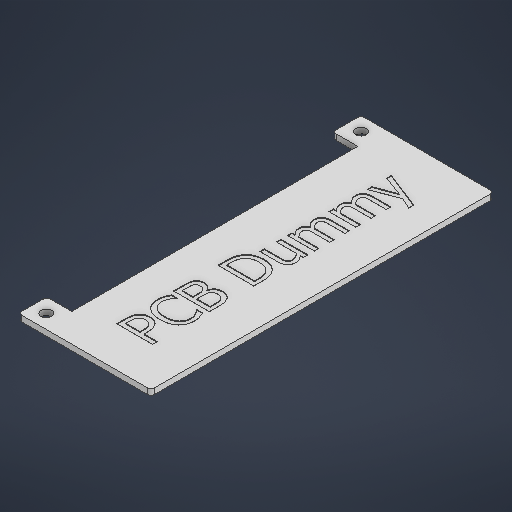
# Autodesk Inventor part: PCBDummy
Saved by Autodesk Inventor 2027 (Build 310192000, 192)
## iProperties
Created: 2026-09-26
Part Number: PCBDummy
Material: Všeobecné
Document SubType Name: Modeling
Designer: Vadim
Density: 1 g/cm^3
Appearance: Výchozí
Author: Vadim
Autodesk Inventor part; units mm, degrees
ref_plane "YZ Plane" through (0, 0, 0) normal (1, 0, 0) x (0, 1, 0)
ref_plane "XZ Plane" through (0, 0, 0) normal (0, 1, 0) x (-1, 0, 0)
ref_plane "XY Plane" through (0, 0, 0) normal (0, 0, 1) x (1, 0, 0)
sketch "Náčrt1" plane through (0, 0, 0) normal (0, 1, 0) x (-1, 0, 0)
  circle A0 centre (3.1, 43.9) radius 1.5
  circle A1 centre (3.1, -43.9) radius 1.5
  line L0 (7, 46.8) -> (7, 40.9)
  line L1 (6, 39.9) -> (0, 39.9)
  line L2 (0, 39.9) -> (0, -39.9)
  line L3 (0, -39.9) -> (6, -39.9)
  line L4 (7, -40.9) -> (7, -46.8)
  line L5 (6, -47.8) -> (-29, -47.8)
  line L6 (-30, -46.8) -> (-30, 46.8)
  line L7 (-29, 47.8) -> (6, 47.8)
  arc A2 (7, 46.8) -> (6, 47.8) centre (6, 46.8) ccw
  arc A3 (6, -47.8) -> (7, -46.8) centre (6, -46.8) ccw
  arc A4 (7, -40.9) -> (6, -39.9) centre (6, -40.9) ccw
  arc A5 (6, 39.9) -> (7, 40.9) centre (6, 40.9) ccw
  line L8 (0, 0) -> (-30, 0)
  arc A6 (-29, 47.8) -> (-30, 46.8) centre (-29, 46.8) ccw
  arc A7 (-30, -46.8) -> (-29, -47.8) centre (-29, -46.8) ccw
  dimension "d1" = 3
  dimension "d2" = 3
  dimension "d3" = 3.9
  dimension "d4" = 3.9
  dimension "d5" = 4
  dimension "d6" = 3.9
  dimension "d7" = 3.9
  dimension "d8" = 4
  dimension "d9" = 1
  dimension "d10" = 87.8
  dimension "d11" = 37
  dimension "d12" = 1
  dimension "d19" = 30
  constraints: 18 end point, 12 point on circle, 12 tangent, 8 centre point, 6 perpendicular, 4 equal radius, 2 midpoint, 1 coincident, 1 collinear
  measures "d1" diameter of A0
  measures "d2" diameter of A1
  measures "d3" distance from line of L0 A0.centre
  measures "d4" distance from line of L7 A0.centre
  measures "d5" distance from line of L1 A0.centre
  measures "d6" distance from line of L4 A1.centre
  measures "d7" distance from line of L5 A1.centre
  measures "d8" distance from line of A1.centre L3
  measures "d9" radius of A2
  measures "d10" distance of A1.centre A0.centre
  measures "d11" distance between parallel lines of L6 L4
  measures "d12" radius of A6
  measures "d19" distance between parallel lines of L6 L2
extrude "Vysunutí1" add sketch "Náčrt1" along normal blind 1.6
sketch "Náčrt2" plane through (0, 1.6, 0) normal (0, 1, 0) x (1, 0, 0)
  arc A0 (-6, -39.9) -> (-7, -40.9) centre (-6, -40.9) ccw projected
  line L0 (-7, -40.9) -> (-7, -46.8) projected
  arc A1 (-7, -46.8) -> (-6, -47.8) centre (-6, -46.8) ccw projected
  line L1 (-6, -47.8) -> (29, -47.8) projected
  arc A2 (29, -47.8) -> (30, -46.8) centre (29, -46.8) ccw projected
  line L2 (30, -46.8) -> (30, 46.8) projected
  arc A3 (30, 46.8) -> (29, 47.8) centre (29, 46.8) ccw projected
  line L3 (29, 47.8) -> (-6, 47.8) projected
  arc A4 (-6, 47.8) -> (-7, 46.8) centre (-6, 46.8) ccw projected
  line L4 (-7, 46.8) -> (-7, 40.9) projected
  arc A5 (-7, 40.9) -> (-6, 39.9) centre (-6, 40.9) ccw projected
  line L5 (-6, 39.9) -> (0, 39.9) projected
  line L6 (0, 39.9) -> (0, -39.9) projected
  line L7 (0, -39.9) -> (-6, -39.9) projected
  circle A6 centre (-3.1, 43.9) radius 1.5 projected
  circle A7 centre (-3.1, -43.9) radius 1.5 projected
  line L8 (1, -37.8) -> (1, 37.8) construction
  line L9 (1, 37.8) -> (22, 37.8) construction
  line L10 (22, 37.8) -> (22, -37.8) construction
  line L11 (22, -37.8) -> (1, -37.8) construction
  line L12 (0, 0) -> (30, 0) construction
  line L13 (11.5, -47.8) -> (11.5, 47.8) construction
  spline S0 degree 2 poles (12.2512, -30.2553) (12.8995, -30.2553) (14.0665, -30.7172) (14.4716, -31.1305) knots 0 0 0 1 2 2 2
  spline S1 degree 2 poles (14.4716, -31.1305) (14.9822, -31.6491) (15.5089, -33.0511) (15.5089, -34.1207) knots 0 0 0 1 2 2 2
  line L14 (15.5089, -34.1207) -> (15.5089, -35.2472)
  line L15 (15.5089, -35.2472) -> (19.2366, -35.2472)
  line L16 (19.2366, -35.2472) -> (19.2366, -36.5762)
  line L17 (19.2366, -36.5762) -> (9.2366, -36.5762)
  line L18 (9.2366, -36.5762) -> (9.2366, -34.064)
  spline S2 degree 2 poles (9.2366, -34.064) (9.2366, -33.1726) (9.5284, -31.9246) (9.8606, -31.4465) knots 0 0 0 1 2 2 2
  spline S3 degree 2 poles (9.8606, -31.4465) (10.2415, -30.8874) (11.4165, -30.2553) (12.2512, -30.2553) knots 0 0 0 1 2 2 2
  spline S4 degree 2 poles (12.2917, -31.641) (11.7731, -31.641) (11.0113, -31.9976) (10.7682, -32.3622) knots 0 0 0 1 2 2 2
  spline S5 degree 2 poles (10.7682, -32.3622) (10.5575, -32.6783) (10.3874, -33.5211) (10.3874, -34.1451) knots 0 0 0 1 2 2 2
  line L19 (10.3874, -34.1451) -> (10.3874, -35.2472)
  line L20 (10.3874, -35.2472) -> (14.3744, -35.2472)
  line L21 (14.3744, -35.2472) -> (14.3744, -34.3395)
  spline S6 degree 2 poles (14.3744, -34.3395) (14.3744, -33.5292) (14.1151, -32.5324) (13.7747, -32.2083) knots 0 0 0 1 2 2 2
  spline S7 degree 2 poles (13.7747, -32.2083) (13.4749, -31.9084) (12.7699, -31.641) (12.2917, -31.641) knots 0 0 0 1 2 2 2
  spline S8 degree 2 poles (19.4149, -25.0851) (19.4149, -26.0575) (18.7585, -27.7026) (18.1021, -28.3023) knots 0 0 0 1 2 2 2
  spline S9 degree 2 poles (18.1021, -28.3023) (17.4538, -28.9019) (15.5089, -29.5583) (14.2447, -29.5583) knots 0 0 0 1 2 2 2
  spline S10 degree 2 poles (14.2447, -29.5583) (12.9887, -29.5583) (11.1248, -28.9182) (10.436, -28.3104) knots 0 0 0 1 2 2 2
  spline S11 degree 2 poles (10.436, -28.3104) (9.7634, -27.7107) (9.0583, -26.0737) (9.0583, -25.0608) knots 0 0 0 1 2 2 2
  spline S12 degree 2 poles (9.0583, -25.0608) (9.0583, -24.5583) (9.2042, -23.675) (9.3177, -23.3023) knots 0 0 0 1 2 2 2
  spline S13 degree 2 poles (9.3177, -23.3023) (9.423, -22.9781) (9.7229, -22.3055) (9.9011, -21.9733) knots 0 0 0 1 2 2 2
  line L22 (9.9011, -21.9733) -> (11.5057, -21.9733)
  line L23 (11.5057, -21.9733) -> (11.5057, -22.0786)
  spline S14 degree 2 poles (11.5057, -22.0786) (11.3436, -22.2569) (10.8898, -22.8079) (10.671, -23.205) knots 0 0 0 1 2 2 2
  spline S15 degree 2 poles (10.671, -23.205) (10.4603, -23.5859) (10.1929, -24.4854) (10.1929, -25.0689) knots 0 0 0 1 2 2 2
  spline S16 degree 2 poles (10.1929, -25.0689) (10.1929, -25.7091) (10.7196, -26.8517) (11.222, -27.2812) knots 0 0 0 1 2 2 2
  spline S17 degree 2 poles (11.222, -27.2812) (11.7326, -27.7026) (13.2804, -28.1726) (14.2447, -28.1726) knots 0 0 0 1 2 2 2
  spline S18 degree 2 poles (14.2447, -28.1726) (15.2739, -28.1726) (16.7569, -27.6783) (17.2674, -27.2488) knots 0 0 0 1 2 2 2
  spline S19 degree 2 poles (17.2674, -27.2488) (17.7618, -26.8274) (18.2642, -25.701) (18.2642, -25.0689) knots 0 0 0 1 2 2 2
  spline S20 degree 2 poles (18.2642, -25.0689) (18.2642, -24.4935) (17.9806, -23.513) (17.7699, -23.1321) knots 0 0 0 1 2 2 2
  spline S21 degree 2 poles (17.7699, -23.1321) (17.5592, -22.7674) (17.1216, -22.2245) (16.9676, -22.0705) knots 0 0 0 1 2 2 2
  line L24 (16.9676, -22.0705) -> (16.9676, -21.9733)
  line L25 (16.9676, -21.9733) -> (18.5559, -21.9733)
  spline S22 degree 2 poles (18.5559, -21.9733) (18.7099, -22.3055) (18.9935, -22.889) (19.1232, -23.3023) knots 0 0 0 1 2 2 2
  spline S23 degree 2 poles (19.1232, -23.3023) (19.269, -23.7399) (19.4149, -24.4854) (19.4149, -25.0851) knots 0 0 0 1 2 2 2
  spline S24 degree 2 poles (16.1653, -13.9506) (16.9109, -13.9506) (18.0535, -14.5178) (18.4263, -14.9878) knots 0 0 0 1 2 2 2
  spline S25 degree 2 poles (18.4263, -14.9878) (18.8639, -15.5551) (19.2366, -16.8436) (19.2366, -17.8647) knots 0 0 0 1 2 2 2
  line L26 (19.2366, -17.8647) -> (19.2366, -20.7334)
  line L27 (19.2366, -20.7334) -> (9.2366, -20.7334)
  line L28 (9.2366, -20.7334) -> (9.2366, -18.0835)
  spline S26 degree 2 poles (9.2366, -18.0835) (9.2366, -17.0138) (9.3744, -15.9441) (9.6418, -15.4579) knots 0 0 0 1 2 2 2
  spline S27 degree 2 poles (9.6418, -15.4579) (9.9254, -14.9149) (10.8574, -14.4206) (11.4895, -14.4206) knots 0 0 0 1 2 2 2
  spline S28 degree 2 poles (11.4895, -14.4206) (12.1945, -14.4206) (13.3128, -15.1661) (13.6288, -15.8225) knots 0 0 0 1 2 2 2
  line L29 (13.6288, -15.8225) -> (13.6775, -15.8225)
  spline S29 degree 2 poles (13.6775, -15.8225) (13.9206, -14.9311) (15.2091, -13.9506) (16.1653, -13.9506) knots 0 0 0 1 2 2 2
  spline S30 degree 2 poles (16.222, -15.3363) (15.6548, -15.3363) (14.9254, -15.6605) (14.6661, -16.1467) knots 0 0 0 1 2 2 2
  spline S31 degree 2 poles (14.6661, -16.1467) (14.5041, -16.4627) (14.4068, -17.2083) (14.4068, -17.8971) knots 0 0 0 1 2 2 2
  line L30 (14.4068, -17.8971) -> (14.4068, -19.4044)
  line L31 (14.4068, -19.4044) -> (18.1021, -19.4044)
  line L32 (18.1021, -19.4044) -> (18.1021, -18.3266)
  spline S32 degree 2 poles (18.1021, -18.3266) (18.1021, -17.4514) (17.94, -16.4465) (17.6807, -16.0575) knots 0 0 0 1 2 2 2
  spline S33 degree 2 poles (17.6807, -16.0575) (17.4133, -15.6848) (16.7488, -15.3363) (16.222, -15.3363) knots 0 0 0 1 2 2 2
  spline S34 degree 2 poles (11.6759, -15.8063) (11.3193, -15.8063) (10.7844, -16.0494) (10.6305, -16.3169) knots 0 0 0 1 2 2 2
  spline S35 degree 2 poles (10.6305, -16.3169) (10.4522, -16.641) (10.3712, -17.4271) (10.3712, -18.1321) knots 0 0 0 1 2 2 2
  line L33 (10.3712, -18.1321) -> (10.3712, -19.4044)
  line L34 (10.3712, -19.4044) -> (13.2966, -19.4044)
  line L35 (13.2966, -19.4044) -> (13.2966, -17.8971)
  spline S36 degree 2 poles (13.2966, -17.8971) (13.2966, -17.2731) (13.1669, -16.6815) (12.9643, -16.3655) knots 0 0 0 1 2 2 2
  spline S37 degree 2 poles (12.9643, -16.3655) (12.7699, -16.0575) (12.1459, -15.8063) (11.6759, -15.8063) knots 0 0 0 1 2 2 2
  spline S38 degree 2 poles (14.2447, -0.4498) (15.6143, -0.4498) (17.8185, -1.56) (18.4344, -2.4919) knots 0 0 0 1 2 2 2
  spline S39 degree 2 poles (18.4344, -2.4919) (18.9125, -3.2536) (19.2366, -4.8177) (19.2366, -6.0332) knots 0 0 0 1 2 2 2
  line L36 (19.2366, -6.0332) -> (19.2366, -8.3347)
  line L37 (19.2366, -8.3347) -> (9.2366, -8.3347)
  line L38 (9.2366, -8.3347) -> (9.2366, -6.0575)
  spline S40 degree 2 poles (9.2366, -6.0575) (9.2366, -4.6475) (9.658, -3.0429) (10.0308, -2.4757) knots 0 0 0 1 2 2 2
  spline S41 degree 2 poles (10.0308, -2.4757) (10.671, -1.5113) (12.7861, -0.4498) (14.2447, -0.4498) knots 0 0 0 1 2 2 2
  spline S42 degree 2 poles (14.2285, -1.8355) (13.0778, -1.8355) (11.4489, -2.5972) (10.987, -3.3509) knots 0 0 0 1 2 2 2
  spline S43 degree 2 poles (10.987, -3.3509) (10.671, -3.8857) (10.3874, -5.0932) (10.3874, -5.9927) knots 0 0 0 1 2 2 2
  line L39 (10.3874, -5.9927) -> (10.3874, -7.0057)
  line L40 (10.3874, -7.0057) -> (18.0859, -7.0057)
  line L41 (18.0859, -7.0057) -> (18.0859, -5.9927)
  spline S44 degree 2 poles (18.0859, -5.9927) (18.0859, -5.1094) (17.8023, -3.7723) (17.4214, -3.2293) knots 0 0 0 1 2 2 2
  spline S45 degree 2 poles (17.4214, -3.2293) (16.9514, -2.5324) (15.3955, -1.8355) (14.2285, -1.8355) knots 0 0 0 1 2 2 2
  line L42 (19.2366, 6.7301) -> (19.2366, 5.466)
  line L43 (19.2366, 5.466) -> (18.41, 5.466)
  spline S46 degree 2 poles (18.41, 5.466) (18.9206, 4.8825) (19.4473, 3.8371) (19.4473, 3.1888) knots 0 0 0 1 2 2 2
  spline S47 degree 2 poles (19.4473, 3.1888) (19.4473, 2.7026) (19.1232, 1.8355) (18.7747, 1.5195) knots 0 0 0 1 2 2 2
  spline S48 degree 2 poles (18.7747, 1.5195) (18.4263, 1.1953) (17.3647, 0.8387) (16.6029, 0.8387) knots 0 0 0 1 2 2 2
  line L44 (16.6029, 0.8387) -> (11.7326, 0.8387)
  line L45 (11.7326, 0.8387) -> (11.7326, 2.1029)
  line L46 (11.7326, 2.1029) -> (16.0113, 2.1029)
  spline S49 degree 2 poles (16.0113, 2.1029) (16.611, 2.1029) (17.3971, 2.1921) (17.6888, 2.346) knots 0 0 0 1 2 2 2
  spline S50 degree 2 poles (17.6888, 2.346) (17.9806, 2.5) (18.248, 3.0267) (18.248, 3.5211) knots 0 0 0 1 2 2 2
  spline S51 degree 2 poles (18.248, 3.5211) (18.248, 3.983) (17.7212, 5.0284) (17.3404, 5.466) knots 0 0 0 1 2 2 2
  line L47 (17.3404, 5.466) -> (11.7326, 5.466)
  line L48 (11.7326, 5.466) -> (11.7326, 6.7301)
  line L49 (11.7326, 6.7301) -> (19.2366, 6.7301)
  line L50 (19.2366, 17.0705) -> (14.893, 17.0705)
  spline S52 degree 2 poles (14.893, 17.0705) (14.3744, 17.0705) (13.4911, 16.9895) (13.248, 16.8598) knots 0 0 0 1 2 2 2
  spline S53 degree 2 poles (13.248, 16.8598) (12.9806, 16.7301) (12.7212, 16.2358) (12.7212, 15.8063) knots 0 0 0 1 2 2 2
  spline S54 degree 2 poles (12.7212, 15.8063) (12.7212, 15.4173) (13.1994, 14.5259) (13.6532, 14.0559) knots 0 0 0 1 2 2 2
  spline S55 degree 2 poles (13.6532, 14.0559) (13.7666, 14.064) (14.0827, 14.0802) (14.2934, 14.0802) knots 0 0 0 1 2 2 2
  line L51 (14.2934, 14.0802) -> (19.2366, 14.0802)
  line L52 (19.2366, 14.0802) -> (19.2366, 12.816)
  line L53 (19.2366, 12.816) -> (14.893, 12.816)
  spline S56 degree 2 poles (14.893, 12.816) (14.3744, 12.816) (13.4911, 12.735) (13.248, 12.6053) knots 0 0 0 1 2 2 2
  spline S57 degree 2 poles (13.248, 12.6053) (12.9806, 12.4757) (12.7212, 11.9814) (12.7212, 11.5519) knots 0 0 0 1 2 2 2
  spline S58 degree 2 poles (12.7212, 11.5519) (12.7212, 11.1467) (13.2318, 10.2472) (13.6288, 9.8258) knots 0 0 0 1 2 2 2
  line L54 (13.6288, 9.8258) -> (19.2366, 9.8258)
  line L55 (19.2366, 9.8258) -> (19.2366, 8.5616)
  line L56 (19.2366, 8.5616) -> (11.7326, 8.5616)
  line L57 (11.7326, 8.5616) -> (11.7326, 9.8258)
  line L58 (11.7326, 9.8258) -> (12.5592, 9.8258)
  spline S59 degree 2 poles (12.5592, 9.8258) (12.0648, 10.3201) (11.5219, 11.2925) (11.5219, 11.876) knots 0 0 0 1 2 2 2
  spline S60 degree 2 poles (11.5219, 11.876) (11.5219, 12.5405) (12.1297, 13.5697) (12.8185, 13.8371) knots 0 0 0 1 2 2 2
  spline S61 degree 2 poles (12.8185, 13.8371) (12.1783, 14.4125) (11.5219, 15.4984) (11.5219, 16.1305) knots 0 0 0 1 2 2 2
  spline S62 degree 2 poles (11.5219, 16.1305) (11.5219, 16.6167) (11.8217, 17.4109) (12.1621, 17.7026) knots 0 0 0 1 2 2 2
  spline S63 degree 2 poles (12.1621, 17.7026) (12.5024, 18.0024) (13.5235, 18.3347) (14.2934, 18.3347) knots 0 0 0 1 2 2 2
  line L59 (14.2934, 18.3347) -> (19.2366, 18.3347)
  line L60 (19.2366, 18.3347) -> (19.2366, 17.0705)
  line L61 (19.2366, 28.6183) -> (14.893, 28.6183)
  spline S64 degree 2 poles (14.893, 28.6183) (14.3744, 28.6183) (13.4911, 28.5373) (13.248, 28.4076) knots 0 0 0 1 2 2 2
  spline S65 degree 2 poles (13.248, 28.4076) (12.9806, 28.278) (12.7212, 27.7836) (12.7212, 27.3541) knots 0 0 0 1 2 2 2
  spline S66 degree 2 poles (12.7212, 27.3541) (12.7212, 26.9652) (13.1994, 26.0737) (13.6532, 25.6037) knots 0 0 0 1 2 2 2
  spline S67 degree 2 poles (13.6532, 25.6037) (13.7666, 25.6118) (14.0827, 25.628) (14.2934, 25.628) knots 0 0 0 1 2 2 2
  line L62 (14.2934, 25.628) -> (19.2366, 25.628)
  line L63 (19.2366, 25.628) -> (19.2366, 24.3639)
  line L64 (19.2366, 24.3639) -> (14.893, 24.3639)
  spline S68 degree 2 poles (14.893, 24.3639) (14.3744, 24.3639) (13.4911, 24.2828) (13.248, 24.1532) knots 0 0 0 1 2 2 2
  spline S69 degree 2 poles (13.248, 24.1532) (12.9806, 24.0235) (12.7212, 23.5292) (12.7212, 23.0997) knots 0 0 0 1 2 2 2
  spline S70 degree 2 poles (12.7212, 23.0997) (12.7212, 22.6945) (13.2318, 21.795) (13.6288, 21.3736) knots 0 0 0 1 2 2 2
  line L65 (13.6288, 21.3736) -> (19.2366, 21.3736)
  line L66 (19.2366, 21.3736) -> (19.2366, 20.1094)
  line L67 (19.2366, 20.1094) -> (11.7326, 20.1094)
  line L68 (11.7326, 20.1094) -> (11.7326, 21.3736)
  line L69 (11.7326, 21.3736) -> (12.5592, 21.3736)
  spline S71 degree 2 poles (12.5592, 21.3736) (12.0648, 21.8679) (11.5219, 22.8404) (11.5219, 23.4238) knots 0 0 0 1 2 2 2
  spline S72 degree 2 poles (11.5219, 23.4238) (11.5219, 24.0883) (12.1297, 25.1175) (12.8185, 25.3849) knots 0 0 0 1 2 2 2
  spline S73 degree 2 poles (12.8185, 25.3849) (12.1783, 25.9603) (11.5219, 27.0462) (11.5219, 27.6783) knots 0 0 0 1 2 2 2
  spline S74 degree 2 poles (11.5219, 27.6783) (11.5219, 28.1645) (11.8217, 28.9587) (12.1621, 29.2504) knots 0 0 0 1 2 2 2
  spline S75 degree 2 poles (12.1621, 29.2504) (12.5024, 29.5502) (13.5235, 29.8825) (14.2934, 29.8825) knots 0 0 0 1 2 2 2
  line L70 (14.2934, 29.8825) -> (19.2366, 29.8825)
  line L71 (19.2366, 29.8825) -> (19.2366, 28.6183)
  line L72 (11.7326, 37.5486) -> (22, 33.513)
  line L73 (22, 33.513) -> (22, 32.1596)
  line L74 (22, 32.1596) -> (18.872, 33.5049)
  line L75 (18.872, 33.5049) -> (11.7326, 30.782)
  line L76 (11.7326, 30.782) -> (11.7326, 32.1434)
  line L77 (11.7326, 32.1434) -> (17.2917, 34.1937)
  line L78 (17.2917, 34.1937) -> (11.7326, 36.2358)
  line L79 (11.7326, 36.2358) -> (11.7326, 37.5486)
  dimension "d5" = 4
  dimension "d15" = 10
  dimension "d16" = 8
  constraints: 4 end point, 4 midpoint, 1 perpendicular, 4 other
  measures "d15" distance between parallel lines of L3 L9
  measures "d16" distance between parallel lines of L2 L10
extrude "Vysunutí2" cut sketch "Náčrt2" against normal blind 0.2 contours S0 S1 L14 L15 L16 L17 L18 S2 S3 | S8 S9 S10 S11 S12 S13 L22 L23 S14 S15 S16 S17 S18 S19 S20 S21 L24 L25 S22 S23 | S24 S25 L26 L27 L28 S26 S27 S28 L29 S29 | S38 S39 L36 L37 L38 S40 S41 | L42 L43 S46 S47 S48 L44 L45 L46 S49 S50 S51 L47 L48 L49 | L50 S52 S53 S54 S55 L51 L52 L53 S56 S57 S58 L54 L55 L56 L57 L58 S59 S60 S61 S62 S63 L59 L60 | L61 S64 S65 S66 S67 L62 L63 L64 S68 S69 S70 L65 L66 L67 L68 L69 S71 S72 S73 S74 S75 L70 L71 | L72 L73 L74 L75 L76 L77 L78 L79
equation "\"d4\" = d3"
equation "\"d6\" = d3"
equation "\"d7\" = d3"
